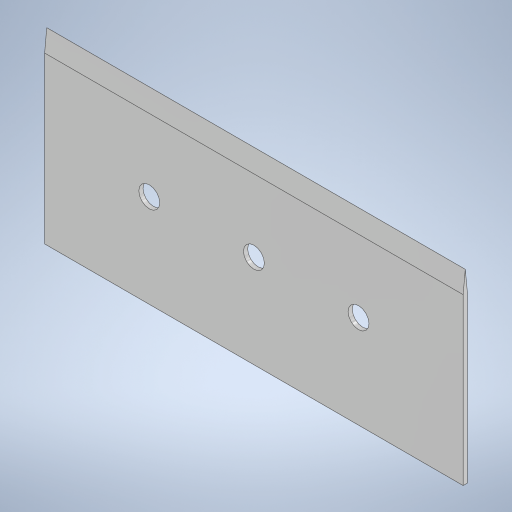
# Autodesk Inventor part: cutter_XB210
Saved by Autodesk Inventor 2024 (Build 280153000, 153)
## iProperties
Created: 2025-03-05
Part Number: cutter_XB210
Material: 鋼 AISI 1015
Document SubType Name: Modeling
Designer: 1412z
Density: 7.87 g/cm^3
Appearance: アルミニウム - つや出し
Author: 1412z
Autodesk Inventor part; units mm, degrees
ref_plane "YZ Plane" through (0, 0, 0) normal (1, 0, 0) x (0, 1, 0)
ref_plane "XZ Plane" through (0, 0, 0) normal (0, 1, 0) x (-1, 0, 0)
ref_plane "XY Plane" through (0, 0, 0) normal (0, 0, 1) x (1, 0, 0)
sketch "スケッチ1" plane through (0, 0, 0) normal (0, 0, 1) x (1, 0, 0)
  line L0 (-20, -8.9) -> (20, -8.9)
  line L1 (20, -8.9) -> (20, 8.9)
  line L2 (20, 8.9) -> (-20, 8.9)
  line L3 (-20, 8.9) -> (-20, -8.9)
  line L4 (-20, -8.9) -> (20, 8.9) construction
  line L5 (20, -8.9) -> (-20, 8.9) construction
  circle A0 centre (0, 0) radius 1
  circle A1 centre (10, 0) radius 1
  circle A2 centre (-10, 0) radius 1
  dimension "d0" = 40
  dimension "d1" = 17.8
  dimension "d2" = 2
  dimension "d3" = 2
  dimension "d4" = 2
  constraints: 12 end point, 3 centre point, 2 midpoint, 2 parallel, 1 coincident, 1 horizontal, 1 perpendicular
  measures "d0" distance of L2.end L1.end
  measures "d1" distance of L1.end L0.end
  measures "d2" diameter of A0
  measures "d3" diameter of A1
  measures "d4" diameter of A2
extrude "押し出し1" add sketch "スケッチ1" along normal blind 0.4
chamfer "面取り1" distance 2 distance2 0.2 1 edges at (0, 8.9, 0.4) measured on face at (0, 8.4, 0.4)
chamfer "面取り2" distance 0.2 distance2 2 1 edges at (0, 8.9, 0) measured on face at (0, 8.9, 0.1)
